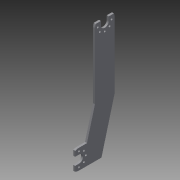
# Autodesk Inventor part: 10
Saved by Autodesk Inventor 2013 (Build 170138000, 138)
## iProperties
Created: 2014-03-10
Material: 一般
Document SubType Name: Modeling
Density: 1 g/cm^3
Designer: andou
Part Number: 10
Author: andou
Title: Dual_Link_Flame(left)
Autodesk Inventor part; units mm, degrees
ref_plane "YZ Plane" through (0, 0, 0) normal (1, 0, 0) x (0, 1, 0)
ref_plane "XZ Plane" through (0, 0, 0) normal (0, 1, 0) x (-1, 0, 0)
ref_plane "XY Plane" through (0, 0, 0) normal (0, 0, 1) x (1, 0, 0)
sketch "スケッチ1" plane through (0, 0, 0) normal (1, 0, 0) x (0, 1, 0)
  line L0 (-20, 60) -> (20, 60)
  line L1 (20, 60) -> (20, -60)
  line L2 (20, -60) -> (-20, -60)
  line L3 (-20, -60) -> (-20, 60)
  point P0 (0, 0)
  dimension "d0" = 120
  dimension "d2" = 40
  dimension "d3" = 20
  dimension "d4" = 60
  constraints: 8 end point, 2 parallel, 1 horizontal, 1 perpendicular
  measures "d0" distance of L2.end L0.start
  measures "d2" distance of L1.end L2.end
  measures "d3" distance from line of L3 point (0, 0)
  measures "d4" distance from line of point (0, 0) L2
extrude "押し出し1" add sketch "スケッチ1" along normal blind 2
sketch "スケッチ3" plane through (0, 0, 0) normal (-1, 0, 0) x (0, 0, 1)
  line L0 (60, -20) -> (60, 20) projected
  line L1 (60, 20) -> (-60, 20) projected
  line L2 (-60, 20) -> (-60, -20) projected
  line L3 (-60, -20) -> (60, -20) projected
  line L4 (-40, -20) -> (-40, -8.0385)
  line L5 (-40, -8.0385) -> (-10, 0)
  line L6 (-10, 0) -> (60, 0)
  line L7 (60, 0) -> (60, 20)
  line L8 (-60, 6.6025) -> (-10, 20)
  point P0 (0, 0)
  dimension "d11" = 20
  dimension "d12" = 15
  dimension "d13" = 15
  dimension "d14" = 20
  dimension "d15" = 120
  dimension "d17" = 70
  dimension "d18" = 70
  constraints: 10 end point, 4 point on line, 3 perpendicular
  measures "d11" distance between parallel lines of L2 L4
  measures "d12" angle of L1 L8
  measures "d13" angle of L6 L5
  measures "d14" distance between parallel lines of L1 L6
  measures "d15" distance between parallel lines of L2 L7
  measures "d17" distance of L7.end L8.end
  measures "d18" distance of L6.end L5.end
extrude "押し出し3" cut sketch "スケッチ3" against normal blind 20 contours L6 L5 L4 L3 L2 L8 L1 L0 keep common part
sketch "スケッチ6" plane through (0, 0, 0) normal (-1, 0, 0) x (0, 0, 1)
  line L0 (-40, -8.0385) -> (-40, -20) projected
  line L1 (-10, 0) -> (-40, -8.0385) projected
  line L2 (60, 0) -> (-10, 0) projected
  line L3 (60, 0) -> (60, 20) projected
  line L4 (60, 20) -> (-10, 20) projected
  line L5 (-60, 6.6025) -> (-10, 20) projected
  line L6 (-60, 6.6025) -> (-60, -20) projected
  line L7 (-60, -20) -> (-40, -20) projected
  arc A0 (-46, -16) -> (-54, -16) centre (-50, -16) ccw
  arc A1 (56, 14) -> (56, 6) centre (56, 10) ccw
  line L8 (-54, -16) -> (-54, -20)
  line L9 (-46, -16) -> (-46, -20)
  line L10 (56, 14) -> (60, 14)
  line L11 (56, 6) -> (60, 6)
  arc A2 (-40.8348, -20) -> (-40, -16) centre (-50, -16) ccw
  arc A3 (-60, -16) -> (-59.1652, -20) centre (-50, -16) ccw
  arc A4 (56, 0) -> (60, 0.8348) centre (56, 10) ccw
  arc A5 (60, 19.1652) -> (56, 20) centre (56, 10) ccw
  point P0 (0, 0)
  dimension "d39" = 8
  dimension "d40" = 4
  dimension "d41" = 4
  dimension "d42" = 10
  dimension "d43" = 10
  constraints: 12 point on circle, 12 point on line, 8 end point, 6 centre point, 6 tangent, 3 equal radius, 3 perpendicular, 2 coincident, 1 parallel
  measures "d39" diameter of A1
  measures "d40" distance from line of A0.centre L7
  measures "d41" distance from line of A1.centre L3
  measures "d42" distance from line of L4 A1.centre
  measures "d43" distance from line of L6 A0.centre
extrude "押し出し6" cut sketch "スケッチ6" against normal blind 11 contours L0 A2 L7 L9 A0 L8 A3 L6 L5 L4 A5 L3 L10 A1 L11 A4 L2 L1 keep common part
sketch "スケッチ7" plane through (0, 0, 0) normal (-1, 0, 0) x (0, 0, 1)
  arc A0 (60, 19.1652) -> (56, 20) centre (56, 10) ccw projected
  arc A1 (-60, -16) -> (-59.1652, -20) centre (-50, -16) ccw projected
  line L0 (-59.1652, -20) -> (-54, -20) projected
  line L1 (60, 0.8348) -> (60, 6) projected
  circle A2 centre (56, 3) radius 1
  circle A3 centre (-57, -16) radius 1
  point P0 (0, 0)
  dimension "d46" = 2
  dimension "d48" = 7
  dimension "d49" = 4
  dimension "d50" = 4
  dimension "d51" = 7
  constraints: 2 centre point, 1 equal radius
  measures "d46" diameter of A2
  measures "d48" distance of A0.centre A2.centre
  measures "d49" distance from line of L1 A2.centre
  measures "d50" distance from line of A3.centre L0
  measures "d51" distance of A1.centre A3.centre
hole "穴1" at (0, -16, -57) at (0, 3, 56) direction (1, 0, 0) diameter 2 end through all
pattern_circular "円形状パターン1" count 5 over 180 about axis through (0, -16, -50) along (1, 0, 0) of "穴1"
pattern_circular "円形状パターン2" count 5 over 180 about axis through (0, 10, 56) along (1, 0, 0) of "穴1"
sketch "スケッチ9" plane through (0, 0, 0) normal (-1, 0, 0) x (0, 0, 1)
  line L0 (56, 20) -> (-10, 20) projected
  line L1 (60, 14) -> (60, 19.1652) projected
  line L2 (10, 20) -> (-10, 20)
  line L3 (-10, 20) -> (-10, 18)
  line L4 (-10, 18) -> (10, 18)
  line L5 (10, 18) -> (10, 20)
  point P0 (0, 0)
  dimension "d85" = 2
  dimension "d87" = 20
  dimension "d88" = 50
  constraints: 8 end point, 2 parallel, 1 horizontal, 1 perpendicular, 1 point on line
  measures "d85" distance between parallel lines of L2 L4
  measures "d87" distance of L3.end L4.end
  measures "d88" distance between parallel lines of L1 L5
extrude "押し出し8" add sketch "スケッチ9" along normal blind 8
sketch "スケッチ10" plane through (0, 20, 56) normal (0, 1, 0) x (1, 0, 0)
  line L0 (0, 66) -> (-8, 66) projected
  line L1 (-8, 46) -> (-8, 66) projected
  circle A0 centre (-3, 51) radius 1
  circle A1 centre (-3, 61) radius 1
  point P0 (0, 56)
  dimension "d94" = 5
  dimension "d95" = 5
  dimension "d96" = 10
  dimension "d97" = 5
  dimension "d98" = 2
  constraints: 2 centre point, 1 equal radius
  measures "d94" distance from line of L1 A1.centre
  measures "d95" distance from line of L1 A0.centre
  measures "d96" distance of A1.centre A0.centre
  measures "d97" distance from line of L0 A1.centre
  measures "d98" diameter of A0
hole "穴3" at (-3, 20, 5) at (-3, 20, -5) direction (0, -1, 0) diameter 2.6 end through all
thread "ねじ5" size "M2.6x0.45" class "6H" standard "ANSI Metric M Profile" full length
thread "ねじ6" size "M2.6x0.45" class "6H" standard "ANSI Metric M Profile" full length
